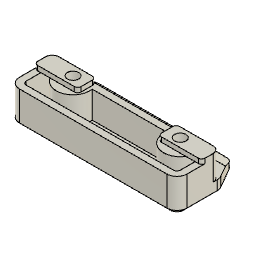
Side Bottom Mid Clip (Autodesk Fusion 360 design; units mm, degrees)
Autodesk Fusion 360 part; units mm, degrees
sketch "Sketch1" plane through (0, 0, 0) normal (0, 0, 1) x (1, 0, 0)
  line L0 (25, 6.4) -> (-25, 6.4)
  line L1 (-25, 6.4) -> (-25, -6.4)
  line L2 (-25, -6.4) -> (25, -6.4)
  line L3 (25, -6.4) -> (25, 6.4)
  line L4 (25, 6.4) -> (-25, -6.4) construction
  line L5 (-25, 6.4) -> (25, -6.4) construction
  line L6 (-16, 3.6) -> (16, 3.6) construction
  line L7 (0, 0) -> (0, 3.6) construction
  circle A0 centre (-16, 3.6) radius 1.7
  circle A1 centre (16, 3.6) radius 1.7
  dimension "d1" = 50
  dimension "d2" = 12.8
  dimension "d4" = 10
  dimension "d5" = 9
  dimension "d6" = 3.4
  constraint horizontal L0
  constraint perpendicular L0 L1
  constraint parallel L0 L2
  constraint parallel L1 L3
  constraint coincident L4 L7.start
  constraint coincident L5 L7.start
  constraint coincident L7.start origin
  constraint horizontal L6
  constraint vertical L7
  constraint midpoint L6 L7.end
  constraint coincident L6.start A0.centre
  constraint coincident L6.end A1.centre
  constraint equal A0 A1
  measures "d1" distance of L1.end L2.end
  measures "d2" distance of L0.end L1.end
  measures "d4" distance of L2 L7.end
  measures "d5" distance of L1 L6.start
  measures "d6" diameter of A0
extrude "Extrude1" add sketch "Sketch1" along normal blind 6
sketch "Sketch2" plane through (0, 0, 0) normal (0, 0, -1) x (1, 0, 0)
  circle A0 centre (-16, -3.6) radius 1.7
  circle A1 centre (16, -3.6) radius 1.7
  line L0 (25, -6.4) -> (25, 6.4)
  line L1 (25, 6.4) -> (-25, 6.4)
  line L2 (-25, 6.4) -> (-25, -6.4)
  line L3 (-25, -6.4) -> (25, -6.4)
  line L4 (25, -6.4) -> (20.3812, -14.4)
  line L5 (20.3812, -14.4) -> (-20.3812, -14.4)
  line L6 (-20.3812, -14.4) -> (-25, -6.4)
  line L7 (0, 0) -> (0, -14.4) construction
  dimension "d9" = 60
  dimension "d10" = 8
  constraint coincident L0.start L3.end
  constraint perpendicular L0 L5
  constraint coincident L2.end L3.start
  constraint coincident L7.start origin
  constraint perpendicular L3 L7
  constraint midpoint L5 L7.end
  measures "d9" angle of L3 L4
  measures "d10" distance of L3 L5
extrude "Extrude2" add sketch "Sketch2" along normal blind 4
sketch "Sketch3" plane through (25, 0, 0) normal (1, 0, 0) x (0, 1, 0)
  line L0 (6.4, 0) -> (6.4, 6)
  line L1 (6.4, 6) -> (-6.4, 6)
  line L2 (-6.4, 6) -> (-6.4, -4)
  line L3 (-6.4, -4) -> (6.4, -4)
  line L4 (6.4, -4) -> (6.4, 0)
  line L5 (14.4, 0) -> (6.4, 0)
  line L6 (6.4, 0) -> (6.4, -4)
  line L7 (6.4, -4) -> (14.4, -4)
  line L8 (14.4, -4) -> (14.4, 0)
  line L9 (10.4, 0) -> (14.4, -1.6)
  dimension "d13" = 1.6
  dimension "d14" = 4
  constraint coincident L5 L9.start
  constraint coincident L8 L9.end
  measures "d13" distance of L5.start L9.end
  measures "d14" distance of L5.start L9.start
extrude "Extrude3" cut sketch "Sketch3" against normal through all contours L5 L8 L9
fillet "Fillet2" radius 2 2 edges at (-25, 6.4, 3) (25, 6.4, 3)
fillet "Fillet1" radius 3 6 edges at (25, -6.4, 1) (-25, -6.4, 1) (-20.3812, 14.4, -2.8) (20.3812, 14.4, -2.8) (-25, 6.4, -2) (25, 6.4, -2)
sketch "Sketch4" plane through (0, 0, -4) normal (0, 0, -1) x (1, 0, 0)
  arc A0 (24.5981, -7.0962) -> (25, -5.5962) centre (22, -5.5962) ccw
  line L0 (25, -5.5962) -> (25, 3.4)
  arc A1 (25, 3.4) -> (22, 6.4) centre (22, 3.4) ccw
  line L1 (22, 6.4) -> (-22, 6.4)
  arc A2 (-22, 6.4) -> (-25, 3.4) centre (-22, 3.4) ccw
  line L2 (-25, 3.4) -> (-25, -5.5962)
  arc A3 (-25, -5.5962) -> (-24.5981, -7.0962) centre (-22, -5.5962) ccw
  line L3 (-24.5981, -7.0962) -> (-21.2472, -12.9)
  arc A4 (-21.2472, -12.9) -> (-18.6491, -14.4) centre (-18.6491, -11.4) ccw
  line L4 (-18.6491, -14.4) -> (18.6491, -14.4)
  arc A5 (18.6491, -14.4) -> (21.2472, -12.9) centre (18.6491, -11.4) ccw
  line L5 (21.2472, -12.9) -> (24.5981, -7.0962)
  circle A6 centre (-16, -3.6) radius 1.7
  circle A7 centre (16, -3.6) radius 1.7
  circle A8 centre (16, -3.6) radius 3
  circle A9 centre (-16, -3.6) radius 3
  dimension "d20" = 6
  constraint concentric A7 A8
  constraint concentric A6 A9
  constraint equal A8 A9
  measures "d20" diameter of A8
extrude "Extrude4" cut sketch "Sketch4" against normal up to surface (3 mm away) contours A8 | A9
chamfer "Chamfer1" distance 1.2 angle 45 12 edges at (-20.1491, 13.9981, -4) (-22.9226, 9.9981, -4) (-24.8978, 6.3726, -4) (-25, 1.0981, -4) (-24.1213, -5.5213, -4) (0, -6.4, -4) (24.1213, -5.5213, -4) (25, 1.0981, -4) (24.8978, 6.3726, -4) (22.9226, 9.9981, -4) (20.1491, 13.9981, -4) (0, 14.4, -4)
shell "Shell1" thickness 2 removed faces 1 at (-4.98, -3.5097, 6)
extrude "Extrude5" add 2 faces at (-20.542, 3.9789, 1) (20.542, 3.9789, 1) along direction (0, 0, 1) up to surface end surface through (0, 0, 6) normal (0, 0, 1) offset 0
sketch "Sketch5" plane through (0, 0, -1) normal (0, 0, -1) x (1, 0, 0)
  circle A0 centre (16, -3.6) radius 1.7
  circle A1 centre (16, -3.6) radius 3
  circle A2 centre (-16, -3.6) radius 1.7
  circle A3 centre (-16, -3.6) radius 3
  line L0 (18.4718, -5.3) -> (13.5282, -5.3)
  line L1 (18.4718, -1.9) -> (13.5282, -1.9)
  line L2 (-13.5282, -5.3) -> (-18.4718, -5.3)
  line L3 (-13.5282, -1.9) -> (-18.4718, -1.9)
  constraint coincident A1 L0.start
  constraint coincident A1 L0.end
  constraint horizontal L0
  constraint coincident A1 L1.start
  constraint coincident A1 L1.end
  constraint parallel L0 L1
  constraint coincident A3 L2.start
  constraint coincident A3 L2.end
  constraint parallel L1 L2
  constraint coincident A3 L3.start
  constraint coincident A3 L3.end
  constraint parallel L2 L3
  constraint tangent A0 L1
  constraint tangent A0 L0
  constraint tangent A2 L2
  constraint tangent A2 L3
extrude "Extrude6" add sketch "Sketch5" along normal blind 0.2 contours A1 L1 | A1 L0 | A3 L3 | A3 L2
sketch "Sketch6" plane through (0, 0, -1) normal (0, 0, -1) x (1, 0, 0)
  line L0 (18.4718, -1.9) -> (16, -1.9)
  arc A0 (16, -5.3) -> (16, -1.9) centre (16, -3.6) ccw
  line L1 (16, -5.3) -> (18.4718, -5.3)
  arc A1 (18.4718, -5.3) -> (18.4718, -1.9) centre (16, -3.6) ccw
  line L2 (16, -1.9) -> (13.5282, -1.9)
  arc A2 (13.5282, -1.9) -> (13.5282, -5.3) centre (16, -3.6) ccw
  line L3 (13.5282, -5.3) -> (16, -5.3)
  arc A3 (16, -1.9) -> (16, -5.3) centre (16, -3.6) ccw
  line L4 (-13.5282, -1.9) -> (-16, -1.9)
  arc A4 (-16, -5.3) -> (-16, -1.9) centre (-16, -3.6) ccw
  line L5 (-16, -5.3) -> (-13.5282, -5.3)
  arc A5 (-13.5282, -5.3) -> (-13.5282, -1.9) centre (-16, -3.6) ccw
  line L6 (-16, -1.9) -> (-18.4718, -1.9)
  arc A6 (-18.4718, -1.9) -> (-18.4718, -5.3) centre (-16, -3.6) ccw
  line L7 (-18.4718, -5.3) -> (-16, -5.3)
  arc A7 (-16, -1.9) -> (-16, -5.3) centre (-16, -3.6) ccw
  line L8 (17.7, -5.3) -> (17.7, -1.9)
  line L9 (14.3, -5.3) -> (14.3, -1.9)
  line L10 (-14.3, -5.3) -> (-14.3, -1.9)
  line L11 (-17.7, -5.3) -> (-17.7, -1.9)
  constraint coincident L1 L8.start
  constraint coincident L0 L8.end
  constraint perpendicular L0 L8
  constraint coincident L3 L9.start
  constraint coincident L2 L9.end
  constraint perpendicular L2 L9
  constraint coincident L5 L10.start
  constraint coincident L4 L10.end
  constraint perpendicular L4 L10
  constraint coincident L7 L11.start
  constraint coincident L6 L11.end
  constraint perpendicular L6 L11
  constraint tangent A0 L8
  constraint tangent A3 L9
  constraint tangent A4 L10
  constraint tangent A7 L11
extrude "Extrude7" cut sketch "Sketch6" against normal blind 0.2 contours L0 A0 L8 | L2 A3 L9 | A0 L1 L8 | L3 A3 L9 | L4 A4 L10 | L6 A7 L11 | A4 L5 L10 | L7 A7 L11
sketch "Sketch7" plane through (0, 0, 6) normal (0, 0, 1) x (-1, 0, 0)
  line L0 (23, -4.4) -> (20.9356, -4.4)
  arc A0 (20.9356, -4.4) -> (11.0644, -4.4) centre (16, -3.6) ccw
  line L1 (11.0644, -4.4) -> (-11.0644, -4.4)
  arc A1 (-11.0644, -4.4) -> (-20.9356, -4.4) centre (-16, -3.6) ccw
  line L2 (-20.9356, -4.4) -> (-23, -4.4)
  line L3 (-23, -4.4) -> (-23, 3.4)
  arc A2 (-22, 4.4) -> (-23, 3.4) centre (-22, 3.4) ccw
  line L4 (-22, 4.4) -> (22, 4.4)
  arc A3 (23, 3.4) -> (22, 4.4) centre (22, 3.4) ccw
  line L5 (23, 3.4) -> (23, -4.4)
  circle A4 centre (-16, -3.6) radius 1.7
  circle A5 centre (16, -3.6) radius 1.7
  arc A6 (25, 3.4) -> (22, 6.4) centre (22, 3.4) ccw
  line L6 (22, 6.4) -> (-22, 6.4)
  arc A7 (-22, 6.4) -> (-25, 3.4) centre (-22, 3.4) ccw
  line L7 (-25, 3.4) -> (-25, -4.4)
  arc A8 (-25, -4.4) -> (-23, -6.4) centre (-23, -4.4) ccw
  line L8 (-23, -6.4) -> (23, -6.4)
  arc A9 (23, -6.4) -> (25, -4.4) centre (23, -4.4) ccw
  line L9 (25, -4.4) -> (25, 3.4)
  line L10 (-25, -1) -> (-12, -1)
  line L11 (-12, -1) -> (-12, -6.4)
  line L12 (12, -6.4) -> (12, -1)
  line L13 (12, -1) -> (25, -1)
  dimension "d31" = 5.4
  dimension "d32" = 13
  constraint perpendicular L7 L10
  constraint coincident L8 L11.end
  constraint perpendicular L8 L11
  constraint coincident L8 L12.start
  constraint perpendicular L8 L12
  constraint coincident L9 L13.end
  constraint perpendicular L9 L13
  constraint equal L10 L13
  constraint coincident L7 L10.start
  constraint equal L11 L12
  measures "d31" distance of L10.end L11.end
  measures "d32" distance of L10.start L10.end
extrude "Extrude8" add sketch "Sketch7" along normal blind 1.4 contours L0 A0 L5 L8 A9 L9 L12 L13 | L0 A0 L5 L13 | A1 L2 L3 L7 A8 L8 L10 L11 | A1 L2 L3 L10
fillet "Fillet3" radius 1 6 edges at (-12, 1, 6.7) (-12, 6.4, 6.7) (12, 6.4, 6.7) (12, 1, 6.7) (25, 1, 6.7) (-25, 1, 6.7)
